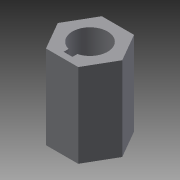
# Autodesk Inventor part: 500 Hex CIM adapter
Saved by Autodesk Inventor 2013 (Build 170138000, 138)
## iProperties
Created: 2013-01-19
Part Number: 500 Hex CIM adapter
Material: Generic
Document SubType Name: Modeling
Designer: actoennies
Density: 1 g/cm^3
Author: actoennies
Autodesk Inventor part; units mm, degrees
ref_plane "YZ Plane" through (0, 0, 0) normal (1, 0, 0) x (0, 1, 0)
ref_plane "XZ Plane" through (0, 0, 0) normal (0, 1, 0) x (-1, 0, 0)
ref_plane "XY Plane" through (0, 0, 0) normal (0, 0, 1) x (1, 0, 0)
sketch "Sketch1" plane through (0, 0, 0) normal (0, 1, 0) x (-1, 0, 0)
  line L0 (3.6662, 6.35) -> (7.3323, 0)
  line L1 (7.3323, 0) -> (3.6662, -6.35)
  line L2 (3.6662, -6.35) -> (-3.6662, -6.35)
  line L3 (-3.6662, -6.35) -> (-7.3323, 0)
  line L4 (-7.3323, 0) -> (-3.6662, 6.35)
  line L5 (-3.6662, 6.35) -> (3.6662, 6.35)
  arc A0 (-1, 3.873) -> (1, 3.873) centre (0, 0) ccw
  line L6 (1, 5) -> (-1, 5)
  line L7 (-1, 5) -> (-1, 3.873)
  line L8 (1, 5) -> (1, 3.873)
  dimension "d0" = 12.7
  dimension "d1" = 8
  dimension "d2" = 2
  dimension "d3" = 1
  dimension "d4" = 5
  constraints: 18 end point, 2 coincident, 2 point on circle, 1 centre point, 1 parallel, 1 perpendicular, 13 other
  measures "d0" distance between parallel lines of L2 L5
  measures "d1" diameter of A0
  measures "d2" distance of L6.start L6.end
  measures "d3" horizontal distance of point (0, 0) L6.start
  measures "d4" distance from line of L6 A0.centre
extrude "Extrusion1" add sketch "Sketch1" along normal blind 19.05
body "Solid1"
